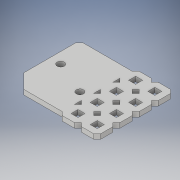
# Autodesk Inventor part: servo mount
Saved by Autodesk Inventor 2017 SP1 (Build 210196100, 196)
## iProperties
Created: 2017-12-11
Part Number: servo mount
Material: Generic
Document SubType Name: Modeling
Designer: rmainhar
Density: 1 g/cm^3
Appearance: Default
Author: rmainhar
Autodesk Inventor part; units mm, degrees
ref_plane "YZ Plane" through (0, 0, 0) normal (1, 0, 0) x (0, 1, 0)
ref_plane "XZ Plane" through (0, 0, 0) normal (0, 1, 0) x (-1, 0, 0)
ref_plane "XY Plane" through (0, 0, 0) normal (0, 0, 1) x (1, 0, 0)
sketch "Sketch1" plane through (0, 0, 0) normal (0, 1, 0) x (-1, 0, 0)
  line L0 (8.138, 0) -> (0, 0)
  line L1 (-2.281, -2.281) -> (0, 0)
  line L2 (-2.281, -2.281) -> (-2.281, -10.419)
  line L3 (0, -12.7) -> (-2.281, -10.419)
  line L4 (-2.281, -14.981) -> (0, -12.7)
  line L5 (-2.281, -14.981) -> (-2.281, -23.119)
  line L6 (0, -25.4) -> (-2.281, -23.119)
  line L7 (-2.281, -27.681) -> (0, -25.4)
  line L8 (-2.281, -27.681) -> (-2.281, -35.819)
  line L9 (0, -38.1) -> (-2.281, -35.819)
  line L10 (-2.281, -40.381) -> (0, -38.1)
  line L11 (-2.281, -40.381) -> (-2.281, -48.519)
  line L12 (0, -50.8) -> (-2.281, -48.519)
  line L13 (-2.281, -53.081) -> (0, -50.8)
  line L14 (-2.281, -53.081) -> (-2.281, -61.219)
  line L15 (0, -63.5) -> (-2.281, -61.219)
  line L16 (-2.281, -65.781) -> (0, -63.5)
  line L17 (-2.281, -65.781) -> (-2.281, -73.919)
  line L18 (0, -76.2) -> (-2.281, -73.919)
  line L19 (-2.281, -78.481) -> (0, -76.2)
  line L20 (-2.281, -78.481) -> (-2.281, -86.619)
  line L21 (0, -88.9) -> (-2.281, -86.619)
  line L22 (-2.281, -91.181) -> (0, -88.9)
  line L23 (-2.281, -91.181) -> (-2.281, -99.319)
  line L24 (0, -101.6) -> (-2.281, -99.319)
  line L25 (-2.281, -103.881) -> (0, -101.6)
  line L26 (-2.281, -103.881) -> (-2.281, -112.019)
  line L27 (0, -114.3) -> (-2.281, -112.019)
  line L28 (-2.281, -116.581) -> (0, -114.3)
  line L29 (-2.281, -116.581) -> (-2.281, -124.719)
  line L30 (0, -127) -> (-2.281, -124.719)
  line L31 (20.838, 0) -> (23.119, -2.281)
  line L32 (20.838, 0) -> (12.7, 0)
  line L33 (10.419, -2.281) -> (12.7, 0)
  line L34 (8.138, 0) -> (10.419, -2.281)
  line L35 (12.7, -12.7) -> (10.419, -10.419)
  line L36 (10.419, -14.981) -> (12.7, -12.7)
  line L37 (8.138, -12.7) -> (10.419, -14.981)
  line L38 (10.419, -10.419) -> (8.138, -12.7)
  line L39 (12.7, -38.1) -> (10.419, -35.819)
  line L40 (10.419, -40.381) -> (12.7, -38.1)
  line L41 (8.138, -38.1) -> (10.419, -40.381)
  line L42 (10.419, -35.819) -> (8.138, -38.1)
  line L43 (12.7, -63.5) -> (10.419, -61.219)
  line L44 (10.419, -65.781) -> (12.7, -63.5)
  line L45 (8.138, -63.5) -> (10.419, -65.781)
  line L46 (10.419, -61.219) -> (8.138, -63.5)
  line L47 (12.7, -88.9) -> (10.419, -86.619)
  line L48 (10.419, -91.181) -> (12.7, -88.9)
  line L49 (8.138, -88.9) -> (10.419, -91.181)
  line L50 (10.419, -86.619) -> (8.138, -88.9)
  line L51 (12.7, -114.3) -> (10.419, -112.019)
  line L52 (10.419, -116.581) -> (12.7, -114.3)
  line L53 (8.138, -114.3) -> (10.419, -116.581)
  line L54 (10.419, -112.019) -> (8.138, -114.3)
  line L55 (20.838, -25.4) -> (23.119, -27.681)
  line L56 (23.119, -23.119) -> (20.838, -25.4)
  line L57 (20.838, -50.8) -> (23.119, -53.081)
  line L58 (23.119, -48.519) -> (20.838, -50.8)
  line L59 (20.838, -76.2) -> (23.119, -78.481)
  line L60 (23.119, -73.919) -> (20.838, -76.2)
  line L61 (20.838, -101.6) -> (23.119, -103.881)
  line L62 (23.119, -99.319) -> (20.838, -101.6)
  line L63 (23.119, -124.719) -> (20.838, -127)
  line L64 (14.4576, -118.3386) -> (14.4576, -122.9614)
  line L65 (19.0804, -118.3386) -> (14.4576, -118.3386)
  line L66 (19.0804, -122.9614) -> (19.0804, -118.3386)
  line L67 (14.4576, -122.9614) -> (19.0804, -122.9614)
  line L68 (14.4576, -105.6386) -> (14.4576, -110.2614)
  line L69 (19.0804, -105.6386) -> (14.4576, -105.6386)
  line L70 (19.0804, -110.2614) -> (19.0804, -105.6386)
  line L71 (14.4576, -110.2614) -> (19.0804, -110.2614)
  line L72 (14.4576, -92.9386) -> (14.4576, -97.5614)
  line L73 (19.0804, -92.9386) -> (14.4576, -92.9386)
  line L74 (19.0804, -97.5614) -> (19.0804, -92.9386)
  line L75 (14.4576, -97.5614) -> (19.0804, -97.5614)
  line L76 (14.4576, -80.2386) -> (14.4576, -84.8614)
  line L77 (19.0804, -80.2386) -> (14.4576, -80.2386)
  line L78 (19.0804, -84.8614) -> (19.0804, -80.2386)
  line L79 (14.4576, -84.8614) -> (19.0804, -84.8614)
  line L80 (14.4576, -67.5386) -> (14.4576, -72.1614)
  line L81 (19.0804, -67.5386) -> (14.4576, -67.5386)
  line L82 (19.0804, -72.1614) -> (19.0804, -67.5386)
  line L83 (14.4576, -72.1614) -> (19.0804, -72.1614)
  line L84 (14.4576, -54.8386) -> (14.4576, -59.4614)
  line L85 (19.0804, -54.8386) -> (14.4576, -54.8386)
  line L86 (19.0804, -59.4614) -> (19.0804, -54.8386)
  line L87 (14.4576, -59.4614) -> (19.0804, -59.4614)
  line L88 (14.4576, -42.1386) -> (14.4576, -46.7614)
  line L89 (19.0804, -42.1386) -> (14.4576, -42.1386)
  line L90 (19.0804, -46.7614) -> (19.0804, -42.1386)
  line L91 (14.4576, -46.7614) -> (19.0804, -46.7614)
  line L92 (14.4576, -29.4386) -> (14.4576, -34.0614)
  line L93 (19.0804, -29.4386) -> (14.4576, -29.4386)
  line L94 (19.0804, -34.0614) -> (19.0804, -29.4386)
  line L95 (14.4576, -34.0614) -> (19.0804, -34.0614)
  line L96 (14.4576, -16.7386) -> (14.4576, -21.3614)
  line L97 (19.0804, -16.7386) -> (14.4576, -16.7386)
  line L98 (19.0804, -21.3614) -> (19.0804, -16.7386)
  line L99 (14.4576, -21.3614) -> (19.0804, -21.3614)
  line L100 (1.7576, -118.3386) -> (1.7576, -122.9614)
  line L101 (6.3804, -118.3386) -> (1.7576, -118.3386)
  line L102 (6.3804, -122.9614) -> (6.3804, -118.3386)
  line L103 (1.7576, -122.9614) -> (6.3804, -122.9614)
  line L104 (1.7576, -105.6386) -> (1.7576, -110.2614)
  line L105 (6.3804, -105.6386) -> (1.7576, -105.6386)
  line L106 (6.3804, -110.2614) -> (6.3804, -105.6386)
  line L107 (1.7576, -110.2614) -> (6.3804, -110.2614)
  line L108 (1.7576, -92.9386) -> (1.7576, -97.5614)
  line L109 (6.3804, -92.9386) -> (1.7576, -92.9386)
  line L110 (6.3804, -97.5614) -> (6.3804, -92.9386)
  line L111 (1.7576, -97.5614) -> (6.3804, -97.5614)
  line L112 (1.7576, -80.2386) -> (1.7576, -84.8614)
  line L113 (6.3804, -80.2386) -> (1.7576, -80.2386)
  line L114 (6.3804, -84.8614) -> (6.3804, -80.2386)
  line L115 (1.7576, -84.8614) -> (6.3804, -84.8614)
  line L116 (1.7576, -67.5386) -> (1.7576, -72.1614)
  line L117 (6.3804, -67.5386) -> (1.7576, -67.5386)
  line L118 (6.3804, -72.1614) -> (6.3804, -67.5386)
  line L119 (1.7576, -72.1614) -> (6.3804, -72.1614)
  line L120 (1.7576, -54.8386) -> (1.7576, -59.4614)
  line L121 (6.3804, -54.8386) -> (1.7576, -54.8386)
  line L122 (6.3804, -59.4614) -> (6.3804, -54.8386)
  line L123 (1.7576, -59.4614) -> (6.3804, -59.4614)
  line L124 (1.7576, -42.1386) -> (1.7576, -46.7614)
  line L125 (6.3804, -42.1386) -> (1.7576, -42.1386)
  line L126 (6.3804, -46.7614) -> (6.3804, -42.1386)
  line L127 (1.7576, -46.7614) -> (6.3804, -46.7614)
  line L128 (1.7576, -29.4386) -> (1.7576, -34.0614)
  line L129 (6.3804, -29.4386) -> (1.7576, -29.4386)
  line L130 (6.3804, -34.0614) -> (6.3804, -29.4386)
  line L131 (1.7576, -34.0614) -> (6.3804, -34.0614)
  line L132 (1.7576, -16.7386) -> (1.7576, -21.3614)
  line L133 (6.3804, -16.7386) -> (1.7576, -16.7386)
  line L134 (6.3804, -21.3614) -> (6.3804, -16.7386)
  line L135 (1.7576, -21.3614) -> (6.3804, -21.3614)
  line L136 (14.4576, -4.0386) -> (14.4576, -8.6614)
  line L137 (19.0804, -4.0386) -> (14.4576, -4.0386)
  line L138 (19.0804, -8.6614) -> (19.0804, -4.0386)
  line L139 (14.4576, -8.6614) -> (19.0804, -8.6614)
  line L140 (1.7576, -4.0386) -> (1.7576, -8.6614)
  line L141 (6.3804, -4.0386) -> (1.7576, -4.0386)
  line L142 (6.3804, -8.6614) -> (6.3804, -4.0386)
  line L143 (1.7576, -8.6614) -> (6.3804, -8.6614)
  line L144 (20.838, -114.3) -> (23.119, -116.581)
  line L145 (23.119, -112.019) -> (20.838, -114.3)
  line L146 (20.838, -88.9) -> (23.119, -91.181)
  line L147 (23.119, -86.619) -> (20.838, -88.9)
  line L148 (20.838, -63.5) -> (23.119, -65.781)
  line L149 (23.119, -61.219) -> (20.838, -63.5)
  line L150 (20.838, -38.1) -> (23.119, -40.381)
  line L151 (23.119, -35.819) -> (20.838, -38.1)
  line L152 (20.838, -12.7) -> (23.119, -14.981)
  line L153 (23.119, -10.419) -> (20.838, -12.7)
  line L154 (12.7, -127) -> (10.419, -124.719)
  line L155 (10.419, -124.719) -> (8.138, -127)
  line L156 (12.7, -101.6) -> (10.419, -99.319)
  line L157 (10.419, -103.881) -> (12.7, -101.6)
  line L158 (8.138, -101.6) -> (10.419, -103.881)
  line L159 (10.419, -99.319) -> (8.138, -101.6)
  line L160 (12.7, -76.2) -> (10.419, -73.919)
  line L161 (10.419, -78.481) -> (12.7, -76.2)
  line L162 (8.138, -76.2) -> (10.419, -78.481)
  line L163 (10.419, -73.919) -> (8.138, -76.2)
  line L164 (12.7, -50.8) -> (10.419, -48.519)
  line L165 (10.419, -53.081) -> (12.7, -50.8)
  line L166 (8.138, -50.8) -> (10.419, -53.081)
  line L167 (10.419, -48.519) -> (8.138, -50.8)
  line L168 (12.7, -25.4) -> (10.419, -23.119)
  line L169 (10.419, -27.681) -> (12.7, -25.4)
  line L170 (8.138, -25.4) -> (10.419, -27.681)
  line L171 (10.419, -23.119) -> (8.138, -25.4)
  line L172 (23.119, -2.281) -> (23.119, -10.419)
  line L173 (23.119, -14.981) -> (23.119, -23.119)
  line L174 (23.119, -27.681) -> (23.119, -35.819)
  line L175 (23.119, -40.381) -> (23.119, -48.519)
  line L176 (23.119, -53.081) -> (23.119, -61.219)
  line L177 (23.119, -65.781) -> (23.119, -73.919)
  line L178 (20.838, -127) -> (12.7, -127)
  line L179 (8.138, -127) -> (0, -127)
  line L180 (23.119, -116.581) -> (23.119, -124.719)
  line L181 (23.119, -103.881) -> (23.119, -112.019)
  line L182 (23.119, -78.481) -> (23.119, -86.619)
  line L183 (23.119, -91.181) -> (23.119, -99.319)
  point P0 (21.9785, -102.7405)
  point P1 (23.119, -107.95)
  point P2 (4.069, -118.3386)
  point P3 (-1.1405, -115.4405)
  point P4 (9.2785, -113.1595)
  dimension "d0" = 12.7
  constraints: 368 end point, 21 vertical, 10 horizontal, 8 perpendicular, 5 midpoint, 19 other
  measures "d0" distance between parallel lines of L142 L138
extrude "Extrusion1" add sketch "Sketch1" along normal blind 3.175
sketch "Sketch2" plane through (0, 3.175, 0) normal (0, 1, 0) x (1, 0, 0)
  line L0 (-23.119, 10.419) -> (-23.119, 2.281) projected
  line L1 (-23.119, 124.719) -> (-23.119, 116.581) projected
  line L2 (-23.119, 2.281) -> (-58.044, 2.281)
  line L3 (-58.044, 2.281) -> (-58.044, 124.719)
  line L4 (-58.044, 124.719) -> (-23.119, 124.719)
  line L5 (-23.119, 124.719) -> (-23.119, 2.281)
  circle A0 centre (-28.575, 19.426) radius 2.3813
  circle A1 centre (-50.8, 28.951) radius 2.3813
  line L6 (-23.119, 101.6) -> (-58.044, 101.6)
  point P0 (0, 0)
  point P1 (-20.838, 101.6)
  dimension "d3" = 4.7625
  dimension "d4" = 28.575
  dimension "d12" = 17.145
  dimension "d14" = 122.438
  dimension "d15" = 9.525
  dimension "d16" = 4.7625
  dimension "d17" = 22.225
  dimension "d25" = 34.925
  constraints: 10 end point, 2 centre point, 2 parallel, 2 perpendicular, 2 point on line, 1 horizontal
  measures "d3" diameter of A0
  measures "d4" horizontal distance of A0.centre point (0, 0)
  measures "d12" distance from line of L2 A0.centre
  measures "d14" distance of L4.end L0.end
  measures "d15" vertical distance of A1.centre A0.centre
  measures "d16" diameter of A1
  measures "d17" horizontal distance of A1.centre A0.centre
  measures "d25" distance of L0.end L2.end
extrude "Extrusion3" add sketch "Sketch2" against normal up to surface (3.175 mm away) contours L0 L2 L3 L6 L5
chamfer "Chamfer1" distance 9.525 angle 45 1 edges at (-58.044, 1.5875, -2.281)
sketch "Sketch4" plane through (0, 3.175, 0) normal (0, 1, 0) x (1, 0, 0)
  line L0 (-48.519, 2.281) -> (-58.044, 11.806) projected
  line L1 (-48.519, 2.281) -> (-23.119, 2.281) projected
  line L2 (-23.119, 2.281) -> (-20.838, 0) projected
  line L3 (-20.838, 0) -> (-12.7, 0) projected
  line L4 (-12.7, 0) -> (-10.419, 2.281) projected
  line L5 (-10.419, 2.281) -> (-8.138, 0) projected
  line L6 (-8.138, 0) -> (0, 0) projected
  line L7 (0, 0) -> (2.281, 2.281) projected
  line L8 (2.281, 2.281) -> (2.281, 10.419) projected
  line L9 (2.281, 10.419) -> (0, 12.7) projected
  line L10 (0, 12.7) -> (2.281, 14.981) projected
  line L11 (2.281, 14.981) -> (2.281, 23.119) projected
  line L12 (2.281, 23.119) -> (0, 25.4) projected
  line L13 (0, 25.4) -> (2.281, 27.681) projected
  line L14 (2.281, 27.681) -> (2.281, 35.819) projected
  line L15 (2.281, 35.819) -> (0, 38.1) projected
  line L16 (0, 38.1) -> (2.281, 40.381) projected
  line L17 (2.281, 40.381) -> (2.281, 48.519) projected
  line L18 (2.281, 48.519) -> (0, 50.8) projected
  line L19 (0, 50.8) -> (2.281, 53.081) projected
  line L20 (2.281, 53.081) -> (2.281, 61.219) projected
  line L21 (2.281, 61.219) -> (0, 63.5) projected
  line L22 (0, 63.5) -> (2.281, 65.781) projected
  line L23 (2.281, 65.781) -> (2.281, 73.919) projected
  line L24 (2.281, 73.919) -> (0, 76.2) projected
  line L25 (0, 76.2) -> (2.281, 78.481) projected
  line L26 (2.281, 78.481) -> (2.281, 86.619) projected
  line L27 (2.281, 86.619) -> (0, 88.9) projected
  line L28 (0, 88.9) -> (2.281, 91.181) projected
  line L29 (2.281, 91.181) -> (2.281, 99.319) projected
  line L30 (2.281, 99.319) -> (0, 101.6) projected
  line L31 (0, 101.6) -> (2.281, 103.881) projected
  line L32 (2.281, 103.881) -> (2.281, 112.019) projected
  line L33 (2.281, 112.019) -> (0, 114.3) projected
  line L34 (0, 114.3) -> (2.281, 116.581) projected
  line L35 (2.281, 116.581) -> (2.281, 124.719) projected
  line L36 (2.281, 124.719) -> (0, 127) projected
  line L37 (0, 127) -> (-8.138, 127) projected
  line L38 (-8.138, 127) -> (-10.419, 124.719) projected
  line L39 (-10.419, 124.719) -> (-12.7, 127) projected
  line L40 (-12.7, 127) -> (-20.838, 127) projected
  line L41 (-20.838, 127) -> (-23.119, 124.719) projected
  line L42 (-23.119, 124.719) -> (-23.119, 116.581) projected
  line L43 (-23.119, 116.581) -> (-20.838, 114.3) projected
  line L44 (-20.838, 114.3) -> (-23.119, 112.019) projected
  line L45 (-23.119, 112.019) -> (-23.119, 103.881) projected
  line L46 (-23.119, 103.881) -> (-20.838, 101.6) projected
  line L47 (-20.838, 101.6) -> (-23.119, 99.319) projected
  line L48 (-23.119, 99.319) -> (-23.119, 101.6) projected
  line L49 (-23.119, 101.6) -> (-58.044, 101.6) projected
  line L50 (-58.044, 101.6) -> (-58.044, 11.806) projected
  line L51 (-23.119, 10.419) -> (-23.119, 14.981) projected
  line L52 (-23.119, 14.981) -> (-20.838, 12.7) projected
  line L53 (-20.838, 12.7) -> (-23.119, 10.419) projected
  line L54 (-23.119, 23.119) -> (-23.119, 27.681) projected
  line L55 (-23.119, 27.681) -> (-20.838, 25.4) projected
  line L56 (-20.838, 25.4) -> (-23.119, 23.119) projected
  line L57 (-23.119, 35.819) -> (-23.119, 40.381) projected
  line L58 (-23.119, 40.381) -> (-20.838, 38.1) projected
  line L59 (-20.838, 38.1) -> (-23.119, 35.819) projected
  line L60 (-23.119, 48.519) -> (-23.119, 53.081) projected
  line L61 (-23.119, 53.081) -> (-20.838, 50.8) projected
  line L62 (-20.838, 50.8) -> (-23.119, 48.519) projected
  line L63 (-23.119, 61.219) -> (-23.119, 65.781) projected
  line L64 (-23.119, 65.781) -> (-20.838, 63.5) projected
  line L65 (-20.838, 63.5) -> (-23.119, 61.219) projected
  line L66 (-23.119, 73.919) -> (-23.119, 78.481) projected
  line L67 (-23.119, 78.481) -> (-20.838, 76.2) projected
  line L68 (-20.838, 76.2) -> (-23.119, 73.919) projected
  circle A0 centre (-28.575, 19.426) radius 2.3813 projected
  circle A1 centre (-50.8, 28.951) radius 2.3813 projected
  line L69 (-1.7576, 4.0386) -> (-6.3804, 4.0386) projected
  line L70 (-6.3804, 4.0386) -> (-6.3804, 8.6614) projected
  line L71 (-6.3804, 8.6614) -> (-1.7576, 8.6614) projected
  line L72 (-1.7576, 8.6614) -> (-1.7576, 4.0386) projected
  line L73 (-14.4576, 4.0386) -> (-19.0804, 4.0386) projected
  line L74 (-19.0804, 4.0386) -> (-19.0804, 8.6614) projected
  line L75 (-19.0804, 8.6614) -> (-14.4576, 8.6614) projected
  line L76 (-14.4576, 8.6614) -> (-14.4576, 4.0386) projected
  line L77 (-1.7576, 16.7386) -> (-6.3804, 16.7386) projected
  line L78 (-6.3804, 16.7386) -> (-6.3804, 21.3614) projected
  line L79 (-6.3804, 21.3614) -> (-1.7576, 21.3614) projected
  line L80 (-1.7576, 21.3614) -> (-1.7576, 16.7386) projected
  line L81 (-1.7576, 29.4386) -> (-6.3804, 29.4386) projected
  line L82 (-6.3804, 29.4386) -> (-6.3804, 34.0614) projected
  line L83 (-6.3804, 34.0614) -> (-1.7576, 34.0614) projected
  line L84 (-1.7576, 34.0614) -> (-1.7576, 29.4386) projected
  line L85 (-1.7576, 42.1386) -> (-6.3804, 42.1386) projected
  line L86 (-6.3804, 42.1386) -> (-6.3804, 46.7614) projected
  line L87 (-6.3804, 46.7614) -> (-1.7576, 46.7614) projected
  line L88 (-1.7576, 46.7614) -> (-1.7576, 42.1386) projected
  line L89 (-1.7576, 54.8386) -> (-6.3804, 54.8386) projected
  line L90 (-6.3804, 54.8386) -> (-6.3804, 59.4614) projected
  line L91 (-6.3804, 59.4614) -> (-1.7576, 59.4614) projected
  line L92 (-1.7576, 59.4614) -> (-1.7576, 54.8386) projected
  line L93 (-1.7576, 67.5386) -> (-6.3804, 67.5386) projected
  line L94 (-6.3804, 67.5386) -> (-6.3804, 72.1614) projected
  line L95 (-6.3804, 72.1614) -> (-1.7576, 72.1614) projected
  line L96 (-1.7576, 72.1614) -> (-1.7576, 67.5386) projected
  line L97 (-1.7576, 80.2386) -> (-6.3804, 80.2386) projected
  line L98 (-6.3804, 80.2386) -> (-6.3804, 84.8614) projected
  line L99 (-6.3804, 84.8614) -> (-1.7576, 84.8614) projected
  line L100 (-1.7576, 84.8614) -> (-1.7576, 80.2386) projected
  line L101 (-1.7576, 92.9386) -> (-6.3804, 92.9386) projected
  line L102 (-6.3804, 92.9386) -> (-6.3804, 97.5614) projected
  line L103 (-6.3804, 97.5614) -> (-1.7576, 97.5614) projected
  line L104 (-1.7576, 97.5614) -> (-1.7576, 92.9386) projected
  line L105 (-1.7576, 105.6386) -> (-6.3804, 105.6386) projected
  line L106 (-6.3804, 105.6386) -> (-6.3804, 110.2614) projected
  line L107 (-6.3804, 110.2614) -> (-1.7576, 110.2614) projected
  line L108 (-1.7576, 110.2614) -> (-1.7576, 105.6386) projected
  line L109 (-1.7576, 118.3386) -> (-6.3804, 118.3386) projected
  line L110 (-6.3804, 118.3386) -> (-6.3804, 122.9614) projected
  line L111 (-6.3804, 122.9614) -> (-1.7576, 122.9614) projected
  line L112 (-1.7576, 122.9614) -> (-1.7576, 118.3386) projected
  line L113 (-14.4576, 16.7386) -> (-19.0804, 16.7386) projected
  line L114 (-19.0804, 16.7386) -> (-19.0804, 21.3614) projected
  line L115 (-19.0804, 21.3614) -> (-14.4576, 21.3614) projected
  line L116 (-14.4576, 21.3614) -> (-14.4576, 16.7386) projected
  line L117 (-14.4576, 29.4386) -> (-19.0804, 29.4386) projected
  line L118 (-19.0804, 29.4386) -> (-19.0804, 34.0614) projected
  line L119 (-19.0804, 34.0614) -> (-14.4576, 34.0614) projected
  line L120 (-14.4576, 34.0614) -> (-14.4576, 29.4386) projected
  line L121 (-14.4576, 42.1386) -> (-19.0804, 42.1386) projected
  line L122 (-19.0804, 42.1386) -> (-19.0804, 46.7614) projected
  line L123 (-19.0804, 46.7614) -> (-14.4576, 46.7614) projected
  line L124 (-14.4576, 46.7614) -> (-14.4576, 42.1386) projected
  line L125 (-14.4576, 54.8386) -> (-19.0804, 54.8386) projected
  line L126 (-19.0804, 54.8386) -> (-19.0804, 59.4614) projected
  line L127 (-19.0804, 59.4614) -> (-14.4576, 59.4614) projected
  line L128 (-14.4576, 59.4614) -> (-14.4576, 54.8386) projected
  line L129 (-14.4576, 67.5386) -> (-19.0804, 67.5386) projected
  line L130 (-19.0804, 67.5386) -> (-19.0804, 72.1614) projected
  line L131 (-19.0804, 72.1614) -> (-14.4576, 72.1614) projected
  line L132 (-14.4576, 72.1614) -> (-14.4576, 67.5386) projected
  line L133 (-14.4576, 80.2386) -> (-19.0804, 80.2386) projected
  line L134 (-19.0804, 80.2386) -> (-19.0804, 84.8614) projected
  line L135 (-19.0804, 84.8614) -> (-14.4576, 84.8614) projected
  line L136 (-14.4576, 84.8614) -> (-14.4576, 80.2386) projected
  line L137 (-14.4576, 92.9386) -> (-19.0804, 92.9386) projected
  line L138 (-19.0804, 92.9386) -> (-19.0804, 97.5614) projected
  line L139 (-19.0804, 97.5614) -> (-14.4576, 97.5614) projected
  line L140 (-14.4576, 97.5614) -> (-14.4576, 92.9386) projected
  line L141 (-14.4576, 105.6386) -> (-19.0804, 105.6386) projected
  line L142 (-19.0804, 105.6386) -> (-19.0804, 110.2614) projected
  line L143 (-19.0804, 110.2614) -> (-14.4576, 110.2614) projected
  line L144 (-14.4576, 110.2614) -> (-14.4576, 105.6386) projected
  line L145 (-14.4576, 118.3386) -> (-19.0804, 118.3386) projected
  line L146 (-19.0804, 118.3386) -> (-19.0804, 122.9614) projected
  line L147 (-19.0804, 122.9614) -> (-14.4576, 122.9614) projected
  line L148 (-14.4576, 122.9614) -> (-14.4576, 118.3386) projected
  line L149 (-12.7, 25.4) -> (-10.419, 27.681) projected
  line L150 (-10.419, 27.681) -> (-8.138, 25.4) projected
  line L151 (-8.138, 25.4) -> (-10.419, 23.119) projected
  line L152 (-10.419, 23.119) -> (-12.7, 25.4) projected
  line L153 (-12.7, 50.8) -> (-10.419, 53.081) projected
  line L154 (-10.419, 53.081) -> (-8.138, 50.8) projected
  line L155 (-8.138, 50.8) -> (-10.419, 48.519) projected
  line L156 (-10.419, 48.519) -> (-12.7, 50.8) projected
  line L157 (-12.7, 76.2) -> (-10.419, 78.481) projected
  line L158 (-10.419, 78.481) -> (-8.138, 76.2) projected
  line L159 (-8.138, 76.2) -> (-10.419, 73.919) projected
  line L160 (-10.419, 73.919) -> (-12.7, 76.2) projected
  line L161 (-12.7, 101.6) -> (-10.419, 103.881) projected
  line L162 (-10.419, 103.881) -> (-8.138, 101.6) projected
  line L163 (-8.138, 101.6) -> (-10.419, 99.319) projected
  line L164 (-10.419, 99.319) -> (-12.7, 101.6) projected
  line L165 (-12.7, 114.3) -> (-10.419, 116.581) projected
  line L166 (-10.419, 116.581) -> (-8.138, 114.3) projected
  line L167 (-8.138, 114.3) -> (-10.419, 112.019) projected
  line L168 (-10.419, 112.019) -> (-12.7, 114.3) projected
  line L169 (-12.7, 88.9) -> (-10.419, 91.181) projected
  line L170 (-10.419, 91.181) -> (-8.138, 88.9) projected
  line L171 (-8.138, 88.9) -> (-10.419, 86.619) projected
  line L172 (-10.419, 86.619) -> (-12.7, 88.9) projected
  line L173 (-12.7, 63.5) -> (-10.419, 65.781) projected
  line L174 (-10.419, 65.781) -> (-8.138, 63.5) projected
  line L175 (-8.138, 63.5) -> (-10.419, 61.219) projected
  line L176 (-10.419, 61.219) -> (-12.7, 63.5) projected
  line L177 (-12.7, 38.1) -> (-10.419, 40.381) projected
  line L178 (-10.419, 40.381) -> (-8.138, 38.1) projected
  line L179 (-8.138, 38.1) -> (-10.419, 35.819) projected
  line L180 (-10.419, 35.819) -> (-12.7, 38.1) projected
  line L181 (-12.7, 12.7) -> (-10.419, 14.981) projected
  line L182 (-10.419, 14.981) -> (-8.138, 12.7) projected
  line L183 (-8.138, 12.7) -> (-10.419, 10.419) projected
  line L184 (-10.419, 10.419) -> (-12.7, 12.7) projected
  line L185 (-23.119, 86.619) -> (-23.119, 91.181) projected
  line L186 (-23.119, 91.181) -> (-20.838, 88.9) projected
  line L187 (-20.838, 88.9) -> (-23.119, 86.619) projected
  line L188 (-23.119, 48.519) -> (-58.044, 48.519)
  line L189 (-58.044, 101.6) -> (-58.044, 11.806) projected
  line L190 (-58.044, 48.519) -> (-58.044, 142.3543)
  line L191 (-58.044, 142.3543) -> (28.0543, 142.3543)
  line L192 (-20.838, 50.8) -> (-23.119, 48.519) projected
  line L193 (-23.119, 48.519) -> (-20.838, 50.8)
  line L194 (-20.838, 50.8) -> (9.501, 50.8)
  line L195 (9.501, 50.8) -> (28.0543, 142.3543)
  point P0 (0, 101.6)
  constraints: 12 end point, 2 horizontal, 1 perpendicular, 1 point on line, 1 vertical
extrude "Extrusion4" cut sketch "Sketch4" against normal through all contours L50 L49 L48 L47 L46 L45 L44 L43 L42 L41 L40 L39 L38 L37 L36 L35 L34 L33 L32 L31 L30 L29 L28 L27 L26 L25 L24 L23 L22 L21 L20 L19 L194 L154 L153 L61 L60 L188 | L190 L191 L195 L194 L19 L20 L21 L22 L23 L24 L25 L26 L27 L28 L29 L30 L31 L32 L33 L34 L35 L36 L37 L38 L39 L40 L41 L42 L43 L44 L45 L46 L47 L48 L49 | L153 L154 L194
chamfer "Chamfer2" distance 2.54 angle 45 1 edges at (-58.044, 1.5875, -48.519)
equation "\"d16\" = d3"
body "Solid1"
